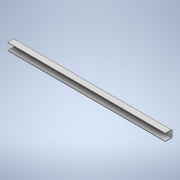
# Autodesk Inventor part: Pieza5
Saved by Autodesk Inventor 2021 (Build 250183000, 183)
## iProperties
Created: 2022-09-12
Part Number: Pieza5
Material: Genérico
Document SubType Name: Modeling
Designer: arthu
Density: 1 g/cm^3
Appearance: Valor por defecto
Author: arthu
Autodesk Inventor part; units mm, degrees
note: some values were not read from the file. Chosen so that the rebuilt part matches the saved one: bend side of "Pieza de plegado2"; bend side of "Pieza de plegado3".
ref_plane "YZ Plane" through (0, 0, 0) normal (1, 0, 0) x (0, 1, 0)
ref_plane "XZ Plane" through (0, 0, 0) normal (0, 1, 0) x (-1, 0, 0)
ref_plane "XY Plane" through (0, 0, 0) normal (0, 0, 1) x (1, 0, 0)
sketch "Boceto2" plane through (0, 0, 0) normal (0, 0, 1) x (1, 0, 0)
  line L0 (490, -50) -> (-510, -50)
  line L1 (-510, -50) -> (-510, 70)
  line L2 (-510, 70) -> (490, 70)
  line L3 (490, 70) -> (490, -50)
  line L4 (-510, 70) -> (-510, 30)
  line L5 (-510, 30) -> (490, 30)
  line L6 (-510, 30) -> (-510, -10)
  line L7 (-510, -10) -> (490, -10)
  point P0 (0, 0)
  dimension "d8" = 1000
  dimension "d14" = 120
  dimension "d15" = 40
  dimension "d16" = 40
  constraints: 16 end point, 4 point on line, 3 perpendicular, 2 parallel, 1 horizontal
  measures "d8" distance of L1.end L2.end
  measures "d14" distance between parallel lines of L0 L2
  measures "d15" distance of L1.end L4.end
  measures "d16" distance of L4.end L6.end
extrude "Extrusión2" add sketch "Boceto2" along normal blind 3
sketch "Boceto4" plane through (0, 0, 3) normal (0, 0, 1) x (1, 0, 0)
  line L0 (-510, 30) -> (490, 30) projected
  line L1 (-510, -10) -> (490, -10) projected
  point P0 (0, 0)
bend part "Pieza de plegado2" radius 3 angle 90 line through (-510, 30, 3) along (1, 0, 0) centre toward (0, 0, 1) moving side (0, 1, 0) both sides yes
sketch "Boceto5" plane through (-510, 27.8787, 3.8787) normal (0, 0.7071068, 0.7071068) x (1, 0, 0)
  line L0 (0, -77.6438) -> (1000, -77.6438) projected
  line L1 (0, -77.6438) -> (0, -37.6438)
  line L2 (0, 0) -> (0, -77.6438) projected
  line L3 (0, -37.6438) -> (1000, -37.6438)
  line L4 (1000, -77.6438) -> (1000, 0) projected
  point P0 (510, -16.9706)
  dimension "d19" = 40
  dimension "d20" = 90
  constraints: 4 end point, 2 point on line
  measures "d19" distance of L0.start L1.end
  measures "d20" angle of L1 L3
bend part "Pieza de plegado3" radius 3 angle 90 line through (-510, 1.2605, 30.4969) along (1, 0, 0) centre toward (0, 0.7071068, 0.7071068) moving side (0, 0.7071068, -0.7071068) both sides yes
